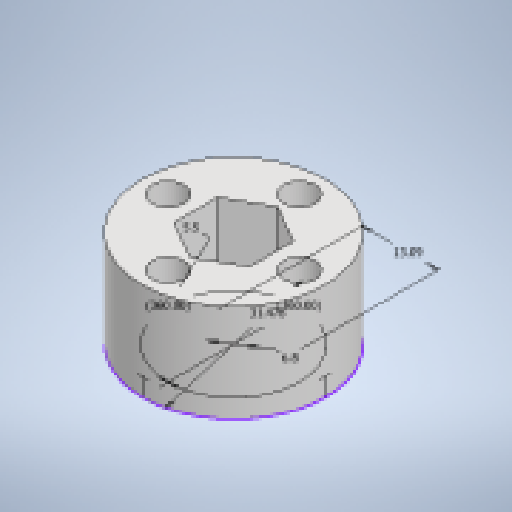
# Autodesk Inventor part: GoBilda Mech Hub 0500 HexV2
Saved by Autodesk Inventor 2023 (Build 270158000, 158)
## iProperties
Created: 2021-12-21
Part Number: GoBilda Mech Hub 0500 HexV2
Material: Generic
Document SubType Name: Modeling
Designer: TakeHomePC
Density: 1 g/cm^3
Appearance: Default
Author: TakeHomePC
Autodesk Inventor part; units mm, degrees
ref_plane "YZ Plane" through (0, 0, 0) normal (1, 0, 0) x (0, 1, 0)
ref_plane "XZ Plane" through (0, 0, 0) normal (0, 1, 0) x (-1, 0, 0)
ref_plane "XY Plane" through (0, 0, 0) normal (0, 0, 1) x (1, 0, 0)
sketch "Sketch1" plane through (0, 0, 0) normal (0, 1, 0) x (-1, 0, 0)
  circle A0 centre (11.3137, 0) radius 2.75
  circle A1 centre (0, 0) radius 15.739
  line L0 (0, -7.5575) -> (-6.545, -3.7788)
  line L1 (-6.545, -3.7788) -> (-6.545, 3.7788)
  line L2 (-6.545, 3.7788) -> (0, 7.5575)
  line L3 (0, 7.5575) -> (6.545, 3.7788)
  line L4 (6.545, 3.7788) -> (6.545, -3.7788)
  line L5 (6.545, -3.7788) -> (0, -7.5575)
  circle A2 centre (0, 11.3137) radius 2.75
  circle A3 centre (-11.3137, 0) radius 2.75
  circle A4 centre (0, -11.3137) radius 2.75
  circle A5 centre (0, 0) radius 3.4
  circle A6 centre (0, -11.3137) radius 4.4253
  circle A7 centre (11.3137, 0) radius 4.4253
  circle A8 centre (0, 11.3137) radius 4.4253
  circle A9 centre (-11.3137, 0) radius 4.4253
  line L6 (-2.8871, -5.8906) -> (-7.481, -13.8474)
  line L7 (-8.2517, -13.4024) -> (-3.6579, -5.4456)
  line L8 (-8.1837, -13.2847) -> (-7.413, -13.7297)
  point P0 (0, 0)
  dimension "d0" = 31.478
  dimension "d3" = 13.09
  dimension "d4" = 5.5
  dimension "d7" = 360
  dimension "d11" = 6.8
  dimension "d14" = 360
  constraints: 18 end point, 10 centre point, 4 coincident, 2 point on line, 31 other
  measures "d0" diameter of A1
  measures "d3" distance between parallel lines of L4 L1
  measures "d4" diameter of A0
  measures "d11" diameter of A5
extrude "Extrusion1" add sketch "Sketch1" along normal blind 16.73 contours L7 L8 L6 A1 | A9 | A1 A8 L2 L1 L0 L7 | L6 L0 A6 A1 | L7 L0 L6 L8 | A7 | A6 L5 L4 L3 A8 A1 | A6 L0 L5 | A8 L3 L2 picked at (-1.3101, -7.6989) picked at (-1.3101, 7.6989)
extrude "Extrusion3" cut sketch "Sketch1" along normal blind 3 contours A0 | A9 | A7 | A6 L0 L5 | A8 L3 L2 | A6 L5 L0 | L2 L3 A8 | A2 | A3 | A4
extrude "Extrusion4" cut sketch "Sketch1" along normal blind 0.5 contours L7 L0 L6 L8
extrude "Extrusion5" cut sketch "Sketch1" along normal through all contours L7 L8 L6 A1
body "Solid1"
